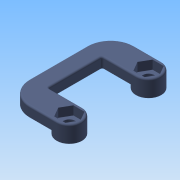
# Autodesk Inventor part: крепление кожуха
Saved by Autodesk Inventor 2017 (Build 210142000, 142)
## iProperties
Part Number: крепление кожуха
Material: Типовые
Document SubType Name: Modeling
Designer: Max
Mass: 0.9629 g
Surface Area: 11.855 cm^2
Volume: 0.9629 cm^3
Density: 1 g/cm^3
Appearance: Резина — синяя
Author: Max
Autodesk Inventor part; units mm, degrees
ref_plane "YZ Plane" through (0, 0, 0) normal (1, 0, 0) x (0, 1, 0)
ref_plane "XZ Plane" through (0, 0, 0) normal (0, 1, 0) x (-1, 0, 0)
ref_plane "XY Plane" through (0, 0, 0) normal (0, 0, 1) x (1, 0, 0)
sketch "Эскиз1" plane through (0, 0, 0) normal (0, 0, 1) x (1, 0, 0)
  line L0 (8.5451, 12.0542) -> (8.5451, 6.2042) construction
  line L1 (8.5451, 6.2042) -> (0.7051, 6.2042) construction
  line L2 (0.7051, 6.2042) -> (0.7051, 12.0542) construction
  line L3 (0.7051, 12.0542) -> (8.5451, 12.0542) construction
  line L4 (16.2451, 0.0542) -> (8.8451, 0.0542) construction
  line L5 (8.8451, 0.0542) -> (8.8451, 5.9042) construction
  line L6 (8.8451, 5.9042) -> (16.2451, 5.9042) construction
  line L7 (16.2451, 5.9042) -> (16.2451, 0.0542) construction
  line L8 (16.2451, 12.0542) -> (16.2451, 6.2042) construction
  line L9 (16.2451, 6.2042) -> (8.8451, 6.2042) construction
  line L10 (8.8451, 6.2042) -> (8.8451, 12.0542) construction
  line L11 (8.8451, 12.0542) -> (16.2451, 12.0542) construction
  line L12 (0.7051, 0.0542) -> (0.7051, 5.9042) construction
  line L13 (0.7051, 5.9042) -> (8.5451, 5.9042) construction
  line L14 (8.5451, 5.9042) -> (8.5451, 0.0542) construction
  line L15 (8.5451, 0.0542) -> (0.7051, 0.0542) construction
  line L16 (15.8851, 27.0542) -> (15.8851, 21.0542) construction
  line L17 (15.8851, 21.0542) -> (2.8851, 21.0542) construction
  line L18 (2.8851, 21.0542) -> (2.8851, 27.0542) construction
  line L19 (2.8851, 27.0542) -> (15.8851, 27.0542) construction
  line L20 (-0.1749, 11.9542) -> (-1.1749, 12.9542) construction
  line L21 (-0.1749, 11.9542) -> (0.2051, 11.9542) construction
  line L22 (0.2051, 11.9542) -> (0.2051, -9.6258) construction
  line L23 (0.2051, -9.6258) -> (-27.4049, -9.6258) construction
  line L24 (-27.4049, -9.6258) -> (-27.4049, -17.1558) construction
  line L25 (-27.4049, -17.1558) -> (10.5451, -17.1558) construction
  line L26 (10.5451, -17.1558) -> (17.0451, -10.6558) construction
  line L27 (17.0451, -10.6558) -> (17.0451, 27.1542) construction
  line L28 (17.0451, 27.1542) -> (-1.1749, 27.1542) construction
  line L29 (-1.1749, 27.1542) -> (-1.1749, 12.9542) construction
  circle A0 centre (10.0951, -7.3458) radius 3 construction
  circle A1 centre (10.0951, 16.1542) radius 3 construction
  circle A2 centre (-24.4049, -14.1558) radius 2 construction
  circle A3 centre (10.0951, 16.1542) radius 1.75
  circle A4 centre (10.0951, -7.3458) radius 1.75
  circle A5 centre (10.0951, 16.1542) radius 3.75
  circle A6 centre (10.0951, -7.3458) radius 3.75
  line L30 (10.0951, 12.4042) -> (0.0951, 12.4042)
  line L31 (0.0951, 12.4042) -> (0.0951, -3.5958)
  line L32 (0.0951, -3.5958) -> (10.0951, -3.5958)
  line L33 (10.0951, -11.0958) -> (-4.9049, -11.0958)
  line L34 (-4.9049, -11.0958) -> (-4.9049, 19.9042)
  line L35 (-4.9049, 19.9042) -> (10.0951, 19.9042)
  point P0 (0, 0)
  dimension "d3" = 3.5
  dimension "d4" = 3.5
  dimension "d5" = 7.5
  dimension "d6" = 7.5
  dimension "d7" = 7.5
  dimension "d8" = 7.5
  dimension "d9" = 10
  dimension "d10" = 5
  constraints: 12 end point, 4 centre point, 4 coincident, 4 point on circle, 4 tangent, 3 perpendicular, 1 parallel
  measures "d3" diameter of A3
  measures "d4" diameter of A4
  measures "d5" diameter of A5
  measures "d6" diameter of A6
  measures "d7" distance between parallel lines of L33 L32
  measures "d8" distance between parallel lines of L30 L35
  measures "d9" distance from line of A1.centre L31
  measures "d10" distance between parallel lines of L34 L31
extrude "Выдавливание1" add sketch "Эскиз1" along normal blind 5
sketch "Эскиз2" plane through (0, 0, 5) normal (0, 0, 1) x (1, 0, 0)
  circle A0 centre (10.0951, 16.1542) radius 1.75 projected
  circle A1 centre (10.0951, -7.3458) radius 1.75 projected
  line L0 (13.386, 16.1542) -> (11.7406, 13.3042)
  line L1 (11.7406, 13.3042) -> (8.4497, 13.3042)
  line L2 (8.4497, 13.3042) -> (6.8042, 16.1542)
  line L3 (6.8042, 16.1542) -> (8.4497, 19.0042)
  line L4 (8.4497, 19.0042) -> (11.7406, 19.0042)
  line L5 (11.7406, 19.0042) -> (13.386, 16.1542)
  line L6 (13.386, -7.3458) -> (11.7406, -10.1958)
  line L7 (11.7406, -10.1958) -> (8.4497, -10.1958)
  line L8 (8.4497, -10.1958) -> (6.8042, -7.3458)
  line L9 (6.8042, -7.3458) -> (8.4497, -4.4958)
  line L10 (8.4497, -4.4958) -> (11.7406, -4.4958)
  line L11 (11.7406, -4.4958) -> (13.386, -7.3458)
  point P0 (0, 0)
  dimension "d13" = 5.7
  dimension "d14" = 5.7
  constraints: 24 end point, 2 coincident, 26 other
  measures "d13" distance between parallel lines of L7 L10
  measures "d14" distance between parallel lines of L1 L4
extrude "Выдавливание2" cut sketch "Эскиз2" against normal blind 2.6
fillet "Сопряжение1" radius 7 2 edges at (-4.9049, 19.9042, 2.5) (-4.9049, -11.0958, 2.5)
fillet "Сопряжение2" radius 0.5 2 edges at (0.0951, 12.4042, 2.5) (0.0951, -3.5958, 2.5)
fillet "Сопряжение3" radius 0.5 12 edges at (-4.9049, 4.4042, 5) (-2.8547, 17.854, 5) (6.0764, 19.9042, 5) (13.8451, 16.1542, 5) (5.3356, 12.4042, 5) (0.2416, 12.2577, 5) (0.0951, 4.4042, 5) (0.2416, -3.4494, 5) (5.3356, -3.5958, 5) (13.8451, -7.3458, 5) (6.0764, -11.0958, 5) (-2.8547, -9.0457, 5)
sketch "Эскиз3" plane through (0, 0, 0) normal (0, 0, -1) x (-1, 0, 0)
  circle A0 centre (-10.0951, -7.3458) radius 1.75 projected
  circle A1 centre (-10.0951, 16.1542) radius 1.75 projected
  arc A2 (-2.0951, -11.0958) -> (4.9049, -4.0958) centre (-2.0951, -4.0958) ccw projected
  line L0 (4.9049, 12.9042) -> (4.9049, -4.0958) projected
  arc A3 (4.9049, 12.9042) -> (-2.0951, 19.9042) centre (-2.0951, 12.9042) ccw projected
  line L1 (-10.0951, 19.9042) -> (-2.0951, 19.9042) projected
  arc A4 (-10.0951, 19.9042) -> (-10.0951, 12.4042) centre (-10.0951, 16.1542) ccw projected
  line L2 (-0.5951, 12.4042) -> (-10.0951, 12.4042) projected
  arc A5 (-0.0951, 11.9042) -> (-0.5951, 12.4042) centre (-0.5951, 11.9042) ccw projected
  line L3 (-0.0951, -3.0958) -> (-0.0951, 11.9042) projected
  arc A6 (-0.5951, -3.5958) -> (-0.0951, -3.0958) centre (-0.5951, -3.0958) ccw projected
  line L4 (-10.0951, -3.5958) -> (-0.5951, -3.5958) projected
  arc A7 (-10.0951, -3.5958) -> (-10.0951, -11.0958) centre (-10.0951, -7.3458) ccw projected
  line L5 (-2.0951, -11.0958) -> (-10.0951, -11.0958) projected
  circle A8 centre (-10.0951, -7.3458) radius 3.75
  circle A9 centre (-10.0951, -7.3458) radius 1.75 projected
  circle A10 centre (-10.0951, -7.3458) radius 1.75
  line L6 (-10.0951, 12.4042) -> (-10.0951, 12.9042) projected
  circle A11 centre (-10.0951, 16.1542) radius 3.75
  point P0 (0, 0)
  dimension "d20" = 3.5
  constraints: 3 coincident, 2 vertical alignment, 1 centre point, 4 other
  measures "d20" diameter of A10
extrude "Выдавливание3" cut sketch "Эскиз3" against normal blind 2 contours L5 A8 L4 A6 L3 A5 L2 A11 L1 A3 L0 A2
